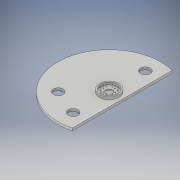
# Autodesk Inventor part: pan_platform
Saved by Autodesk Inventor 2018 (Build 220112000, 112)
## iProperties
Created: 2018-04-14
Part Number: pan_platform
Material: Generic
Document SubType Name: Modeling
Designer: scwu
Density: 1 g/cm^3
Appearance: Default
Author: scwu
Autodesk Inventor part; units mm, degrees
ref_plane "XZ Plane" through (0, 0, 0) normal (0, 1, 0) x (-1, 0, 0)
sketch "Sketch1" plane through (0, 0, 0) normal (0, 1, 0) x (-1, 0, 0)
  circle A0 centre (0, 0) radius 63.5
  circle A1 centre (0, -7.2) radius 0.6
  circle A2 centre (3.5, -7.2) radius 0.6
  circle A3 centre (-3.5, -7.2) radius 0.6
  circle A4 centre (7.2, 3.5) radius 0.6
  circle A5 centre (7.2, 0) radius 0.6
  circle A6 centre (7.2, -3.5) radius 0.6
  circle A7 centre (-3.5, 7.2) radius 0.6
  circle A8 centre (0, 7.2) radius 0.6
  circle A9 centre (3.5, 7.2) radius 0.6
  circle A10 centre (-7.2, -3.5) radius 0.6
  circle A11 centre (-7.2, 0) radius 0.6
  circle A12 centre (-7.2, 3.5) radius 0.6
  circle A13 centre (0, 0) radius 10.4
  circle A14 centre (0, 0) radius 12
  circle A15 centre (0, 0) radius 4
  dimension "d0" = 127
  dimension "d1" = 7.2
  dimension "d2" = 1.2
  dimension "d3" = 3.5
  dimension "d4" = 3.5
  dimension "d5" = 1.2
  dimension "d6" = 1.2
  dimension "d9" = 360
  dimension "d15" = 20.8
  dimension "d16" = 24
  dimension "d19" = 8
  constraints: 16 centre point, 5 coincident, 1 horizontal alignment, 25 other
  measures "d0" diameter of A0
  measures "d1" distance of point (0, -7.2) point (0, 0)
  measures "d2" diameter of A1
  measures "d3" distance of A1.centre point (3.5, -7.2)
  measures "d4" distance of point (-3.5, -7.2) point (0, -7.2)
  measures "d5" diameter of A2
  measures "d6" diameter of A3
  measures "d15" diameter of A13
  measures "d16" diameter of A14
  measures "d19" diameter of A15
extrude "Extrusion1" add sketch "Sketch1" along normal blind 3 contours A0 | A13 | A14
extrude "Extrusion2" add sketch "Sketch1" along normal blind 6 contours A1 | A2 | A3 | A4 | A5 | A6 | A7 | A8 | A9 | A10 | A11 | A12
extrude "Extrusion3" add sketch "Sketch1" along normal blind 6 contours A14
extrude "Extrusion4" add sketch "Sketch1" along normal blind 2 contours A15
sketch "Sketch2" plane through (0, 0, 0) normal (0, -1, 0) x (1, 0, 0)
  line L0 (-17.5, 11.3) -> (-44.5, 11.3) construction
  line L1 (-44.5, 11.3) -> (-44.5, -29.7) construction
  line L2 (-44.5, -29.7) -> (-17.5, -29.7) construction
  line L3 (-17.5, -29.7) -> (-17.5, 11.3) construction
  line L4 (-47.5, 14.3) -> (-47.5, 8.3)
  line L5 (-47.5, 8.3) -> (-44.5, 8.3)
  line L6 (-44.5, 8.3) -> (-44.5, 11.3)
  line L7 (-17.5, 11.3) -> (-17.5, 19.3)
  line L8 (-17.5, 19.3) -> (-20.5, 19.3)
  line L9 (-20.5, 19.3) -> (-20.5, 11.3)
  line L10 (-20.5, 11.3) -> (-17.5, 11.3)
  line L11 (-44.5, -9.2) -> (-17.5, -9.2) construction
  line L12 (-17.5, -29.7) -> (-44.5, -29.7) construction
  line L13 (-44.5, -29.7) -> (-41.5, -29.7)
  line L14 (-41.5, -29.7) -> (-41.5, -32.7)
  line L15 (-41.5, -32.7) -> (-47.5, -32.7)
  line L16 (-47.5, -32.7) -> (-47.5, -26.7)
  line L17 (-47.5, -26.7) -> (-44.5, -26.7)
  line L18 (-44.5, -26.7) -> (-44.5, -29.7)
  line L19 (-17.5, -29.7) -> (-17.5, -37.7)
  line L20 (-17.5, -37.7) -> (-20.5, -37.7)
  line L21 (-20.5, -37.7) -> (-20.5, -29.7)
  line L22 (-20.5, -29.7) -> (-17.5, -29.7)
  line L23 (-47.5, 14.3) -> (-44.5, 14.3)
  line L24 (-44.5, 14.3) -> (-44.5, 11.3)
  point P0 (0, 0)
  point P1 (-41.5, 11.3)
  point P2 (-31, 0)
  dimension "d22" = 27
  dimension "d23" = 41
  dimension "d24" = 3
  dimension "d28" = 6
  dimension "d29" = 3
  dimension "d31" = 8
  dimension "d32" = 3
  dimension "d33" = 8
  dimension "d34" = 90
  dimension "d50" = 44.5
  dimension "d51" = 29.7
  dimension "d52" = 3
  dimension "d53" = 3
  constraints: 50 end point, 7 symmetric about line, 6 perpendicular, 3 parallel, 2 horizontal, 2 midpoint, 2 point on line, 1 horizontal alignment
  measures "d22" distance of L2.end L1.end
  measures "d23" distance of L1.end L0.end
  measures "d24" distance of L0.end point (-41.5, 11.3)
  measures "d28" distance of L4.start L4.end
  measures "d29" distance of L4.end L5.end
  measures "d31" distance of L0.start L7.end
  measures "d32" distance of L7.end L8.end
  measures "d33" distance of L8.end L9.end
  measures "d34" angle of L9 L8
  measures "d50" distance from line of point (0, 0) L1
  measures "d51" distance from line of L2 point (-31, 0)
  measures "d52" distance of L13.end L14.end
  measures "d53" distance of L17.end L1.end
extrude "Extrusion5" add sketch "Sketch2" along normal blind 12 contours L23 L24 L6 L5 L4 | L13 L14 L15 L16 L17 L18
extrude "Extrusion6" add sketch "Sketch2" along normal blind 20 contours L10 L9 L8 L7 | L19 L20 L21 L22
ref_plane "Work Plane1" through (-17.5, 0, -9.2) normal (1, 0, 0) x (0, 0, -1)
sketch "Sketch3" plane through (-17.5, 0, -9.2) normal (1, 0, 0) x (0, 0, -1)
  line L0 (0, 0) -> (0, -20) construction
  line L1 (0, 0) -> (20, 0) construction
  line L2 (28.5, -20) -> (20.5, -20) projected
  line L3 (24.8, -20) -> (24.8, 0) construction
  line L4 (24.8, -10) -> (0, -10) construction
  point P0 (-9.2, 0)
  point P1 (0, 0)
  point P2 (24.8, -15)
  point P3 (24.8, -5)
  point P4 (-24.8, -15)
  point P5 (-24.8, -5)
  dimension "d39" = 20
  dimension "d40" = 90
  dimension "d41" = 24.8
  dimension "d42" = 10
  constraints: 8 end point, 4 symmetric about line, 3 point on line, 2 midpoint, 2 vertical, 1 horizontal, 1 perpendicular
  measures "d39" distance of L0.start L0.end
  measures "d40" angle of L0 L1
  measures "d41" distance between parallel lines of L0 L3
  measures "d42" distance of point (24.8, -5) point (24.8, -15)
hole "Hole1" at (-17.5, -15, 15.6) at (-17.5, -5, 15.6) at (-17.5, -5, -34) at (-17.5, -15, -34) direction (-1, 0, 0) diameter 3 depth 3
sketch "Sketch4" plane through (0, 0, 0) normal (0, -1, 0) x (1, 0, 0)
  point P0 (0, 0)
  point P1 (44.45, 0)
  point P2 (31.4309, 31.4309)
  point P3 (0, 44.45)
  point P4 (-31.4309, 31.4309)
  point P5 (-44.45, 0)
  point P6 (-31.4309, -31.4309)
  point P7 (0, -44.45)
  point P8 (31.4309, -31.4309)
  dimension "d56" = 360
  constraints: 9 other
hole "Hole2" at (-31.4309, 0, 31.4309) at (0, 0, 44.45) at (31.4309, 0, 31.4309) at (44.45, 0, 0) at (31.4309, 0, -31.4309) at (0, 0, -44.45) direction (0, 1, 0) diameter 12 end through all
ref_plane "Work Plane2" through (16, 0, 0) normal (1, 0, 0) x (0, 1, 0)
split "Split1" plane through (16, 0, 0) removes the side toward (1, 0, 0)
body "Solid1"
